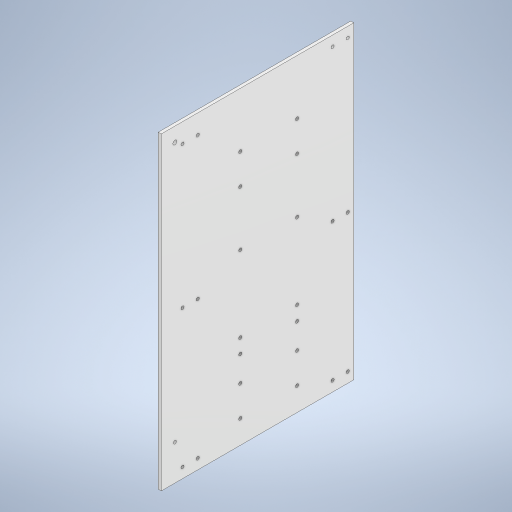
# Autodesk Inventor part: BP_Exterior-Right
Saved by Autodesk Inventor 2024.3 (Build 283343000, 343)
## iProperties
Created: 2025-04-22
Part Number: BP_Exterior-Right
Material: PBT プラスチック
Document SubType Name: Modeling
Designer: ngt-a
Density: 1.31 g/cm^3
Appearance: 滑らか - 白
Mass: 218.125 g
Surface Area: 1149.08 cm^2
Volume: 166.508 cm^3
Author: ngt-a
Autodesk Inventor part; units mm, degrees
ref_plane "YZ Plane" through (0, 0, 0) normal (1, 0, 0) x (0, 1, 0)
ref_plane "XZ Plane" through (0, 0, 0) normal (0, 1, 0) x (-1, 0, 0)
ref_plane "XY Plane" through (0, 0, 0) normal (0, 0, 1) x (1, 0, 0)
sketch "スケッチ1" plane through (0, 0, 0) normal (1, 0, 0) x (0, 1, 0)
  line L0 (75, 87.5) -> (-75, 87.5)
  line L1 (-75, 87.5) -> (-75, -87.5)
  line L2 (-75, -87.5) -> (75, -87.5)
  line L3 (75, -87.5) -> (75, 87.5)
  line L4 (75, 87.5) -> (-75, -87.5) construction
  line L5 (-75, 87.5) -> (75, -87.5) construction
  point P0 (0, 0)
  dimension "d0" = 150
  dimension "d1" = 175
  constraints: 12 end point, 2 midpoint, 2 parallel, 1 horizontal, 1 perpendicular
  measures "d0" distance of L1.end L2.end
  measures "d1" distance of L2.end L0.start
extrude "押し出し1" add sketch "スケッチ1" along normal blind 3
sketch "スケッチ2" plane through (3, 0, 0) normal (1, 0, 0) x (0, 0, -1)
  circle A0 centre (81.5, 66) radius 1.5
  circle A1 centre (66.5, 66) radius 1.5
  line L0 (87.5, -75) -> (87.5, 75) projected
  line L1 (87.5, 75) -> (-87.5, 75) projected
  line L2 (-87.5, 75) -> (-87.5, -75) projected
  line L3 (-87.5, 0) -> (87.5, 0)
  circle A2 centre (66.5, -70) radius 1.5
  circle A3 centre (81.5, -70) radius 1.5
  line L4 (-87.5, -75) -> (87.5, -75) projected
  point P0 (0, 0)
  dimension "d4" = 3
  dimension "d5" = 6
  dimension "d7" = 15
  dimension "d9" = 3
  dimension "d20" = 3
  dimension "d21" = 3
  dimension "d22" = 6
  dimension "d23" = 15
  dimension "d24" = 5
  dimension "d25" = 5
  dimension "d66" = 141
  dimension "d67" = 141
  constraints: 4 centre point, 2 end point, 2 midpoint
  measures "d4" diameter of A0
  measures "d5" distance from line of L0 A0.centre
  measures "d7" distance of A0.centre A1.centre
  measures "d9" diameter of A1
  measures "d20" diameter of A2
  measures "d21" diameter of A3
  measures "d22" distance from line of L0 A3.centre
  measures "d23" distance of A3.centre A2.centre
  measures "d24" distance from line of L4 A3.centre
  measures "d25" distance from line of A2.centre L4
  measures "d66" distance from line of L4 A0.centre
  measures "d67" distance from line of L4 A1.centre
extrude "押し出し2" cut sketch "スケッチ2" against normal through all contours A0 | A1 | A2 | A3
sketch "スケッチ3" plane through (0, 0, 0) normal (-1, 0, 0) x (0, 0, 1)
  circle A0 centre (81.5, 66) radius 1.5
  circle A1 centre (66.5, 66) radius 1.5
  line L0 (87.5, 75) -> (87.5, -75) projected
  line L1 (-87.5, 75) -> (87.5, 75) projected
  line L2 (-87.5, -75) -> (-87.5, 75) projected
  line L3 (-87.5, 0) -> (87.5, 0)
  circle A2 centre (81.5, -70) radius 1.5
  circle A3 centre (66.5, -70) radius 1.5
  line L4 (87.5, -75) -> (-87.5, -75) projected
  point P0 (0, 0)
  dimension "d12" = 6
  dimension "d13" = 3
  dimension "d14" = 15
  dimension "d15" = 3
  dimension "d26" = 3
  dimension "d27" = 3
  dimension "d28" = 15
  dimension "d29" = 6
  dimension "d30" = 5
  dimension "d31" = 5
  dimension "d64" = 141
  dimension "d65" = 141
  constraints: 4 centre point, 2 end point, 2 midpoint
  measures "d12" distance from line of L0 A0.centre
  measures "d13" diameter of A1
  measures "d14" distance of A0.centre A1.centre
  measures "d15" diameter of A0
  measures "d26" diameter of A3
  measures "d27" diameter of A2
  measures "d28" distance of A2.centre A3.centre
  measures "d29" distance from line of L0 A2.centre
  measures "d30" distance from line of L4 A2.centre
  measures "d31" distance from line of L4 A3.centre
  measures "d64" distance from line of L4 A1.centre
  measures "d65" distance from line of L4 A0.centre
sketch "スケッチ6" plane through (3, 0, 0) normal (1, 0, 0) x (0, 0, -1)
  circle A0 centre (-24.5, -57) radius 1.5
  circle A1 centre (31.5, -57) radius 1.5
  circle A2 centre (-24.5, -27) radius 1.5
  circle A3 centre (31.5, -27) radius 1.5
  line L0 (-87.5, -75) -> (87.5, -75) projected
  line L1 (-87.5, 75) -> (-87.5, -75) projected
  line L2 (87.5, -75) -> (87.5, 75) projected
  point P0 (0, 0)
  dimension "d32" = 3
  dimension "d33" = 3
  dimension "d34" = 3
  dimension "d35" = 18
  dimension "d36" = 18
  dimension "d38" = 30
  dimension "d43" = 3
  dimension "d46" = 56
  dimension "d47" = 56
  dimension "d50" = 56
  dimension "d51" = 56
  constraints: 4 centre point
  measures "d32" diameter of A2
  measures "d33" diameter of A0
  measures "d34" diameter of A1
  measures "d35" distance from line of L0 A0.centre
  measures "d36" distance from line of L0 A1.centre
  measures "d38" distance of A1.centre A3.centre
  measures "d43" diameter of A3
  measures "d46" distance of A3.centre A2.centre
  measures "d47" distance of A1.centre A0.centre
  measures "d50" distance from line of L2 A3.centre
  measures "d51" distance from line of L2 A1.centre
extrude "押し出し4" cut sketch "スケッチ6" against normal through all
sketch "スケッチ7" plane through (0, -75, 87.5) normal (0, 0, 1) x (1, 0, 0)
  line L0 (0, 150) -> (3, 150) projected
  line L1 (0, 0) -> (3, 0) projected
  line L2 (0, 150) -> (3, 150)
  line L3 (3, 150) -> (3, 0)
  line L4 (3, 0) -> (0, 0)
  line L5 (0, 0) -> (0, 150)
  point P0 (0, 75)
  constraints: 8 end point, 2 parallel, 1 horizontal, 1 perpendicular
extrude "押し出し5" add sketch "スケッチ7" along normal blind 10
sketch "スケッチ9" plane through (0, -75, -87.5) normal (0, -1, 0) x (1, 0, 0)
  line L0 (3, 0) -> (3, 185) projected
  line L1 (0, 185) -> (0, 0) projected
  line L2 (3, 18) -> (0, 18)
  line L3 (0, 18) -> (0, 43)
  line L4 (0, 43) -> (3, 43)
  line L5 (3, 43) -> (3, 18)
  line L6 (0, 142) -> (3, 142)
  line L7 (3, 142) -> (3, 167)
  line L8 (3, 167) -> (0, 167)
  line L9 (0, 167) -> (0, 142)
  line L10 (0, 0) -> (3, 0) projected
  line L11 (0, 185) -> (3, 185) projected
  point P0 (0, 87.5)
  point P1 (1.5, 185)
  point P2 (0, 167)
  point P3 (3, 142)
  point P4 (3, 43)
  point P5 (0, 18)
  dimension "d58" = 18
  dimension "d59" = 25
  dimension "d60" = 18
  dimension "d61" = 25
  constraints: 16 end point, 4 parallel, 4 point on line, 2 horizontal, 2 perpendicular, 1 midpoint
  measures "d58" distance between parallel lines of L2 L10
  measures "d59" distance between parallel lines of L2 L4
  measures "d60" distance from line of point (1.5, 185) L8
  measures "d61" distance between parallel lines of L8 L6
extrude "押し出し7" add sketch "スケッチ9" along normal blind 5
sketch "スケッチ10" plane through (0, 75, -87.5) normal (0, 1, 0) x (1, 0, 0)
  line L0 (0, 0) -> (0, -185) projected
  line L1 (3, 0) -> (3, -185) projected
  line L2 (0, 0) -> (3, 0)
  line L3 (3, 0) -> (3, -185)
  line L4 (3, -185) -> (0, -185)
  line L5 (0, -185) -> (0, 0)
  point P0 (0, -87.5)
  point P1 (3, 0)
  point P2 (0, -185)
  constraints: 8 end point, 2 parallel, 1 horizontal, 1 perpendicular
extrude "押し出し8" add sketch "スケッチ10" along normal blind 150
sketch "スケッチ11" plane through (3, 0, 0) normal (1, 0, 0) x (0, 0, -1)
  line L0 (44.5, -75) -> (-54.5, -75) projected
  line L1 (-54.5, -75) -> (44.5, -75)
  line L2 (44.5, -75) -> (44.5, -6)
  line L3 (44.5, -6) -> (-54.5, -6)
  line L4 (-54.5, -6) -> (-54.5, -75)
  line L5 (-54.5, -6) -> (44.5, -6)
  line L6 (44.5, -6) -> (44.5, 123)
  line L7 (44.5, 123) -> (-54.5, 123)
  line L8 (-54.5, 123) -> (-54.5, -6)
  circle A0 centre (-24.5, 87) radius 1.5
  circle A1 centre (31.5, 87) radius 1.5
  circle A2 centre (31.5, 12) radius 1.5
  circle A3 centre (-24.5, 12) radius 1.5
  line L9 (-54.5, 123) -> (44.5, 123)
  line L10 (44.5, 123) -> (44.5, 192)
  line L11 (44.5, 192) -> (-54.5, 192)
  line L12 (-54.5, 192) -> (-54.5, 123)
  circle A4 centre (31.5, 141) radius 1.5
  circle A5 centre (-24.5, 141) radius 1.5
  circle A6 centre (-24.5, 171) radius 1.5
  circle A7 centre (31.5, 171) radius 1.5
  point P0 (0, 0)
  point P1 (-5, -75)
  dimension "d70" = 69
  dimension "d71" = 129
  dimension "d72" = 3
  dimension "d73" = 3
  dimension "d74" = 30
  dimension "d75" = 13
  dimension "d89" = 3
  dimension "d90" = 3
  dimension "d136" = 69
  dimension "d137" = 18
  dimension "d138" = 18
  dimension "d139" = 75
  dimension "d140" = 75
  dimension "d141" = 18
  dimension "d142" = 18
  dimension "d143" = 3
  dimension "d144" = 3
  dimension "d145" = 30
  dimension "d146" = 30
  dimension "d147" = 3
  dimension "d148" = 3
  constraints: 24 end point, 8 centre point, 6 parallel, 3 horizontal, 3 perpendicular, 1 midpoint
  measures "d70" distance of L1.end L2.end
  measures "d71" distance of L5.end L6.end
  measures "d72" diameter of A0
  measures "d73" diameter of A1
  measures "d74" distance from line of A0.centre L8
  measures "d75" distance from line of L6 A1.centre
  measures "d89" diameter of A3
  measures "d90" diameter of A2
  measures "d136" distance of L9.end L10.end
  measures "d137" distance from line of L3 A3.centre
  measures "d138" distance from line of L3 A2.centre
  measures "d139" distance of A3.centre A0.centre
  measures "d140" distance of A2.centre A1.centre
  measures "d141" distance from line of L7 A4.centre
  measures "d142" distance from line of L7 A5.centre
  measures "d143" diameter of A5
  measures "d144" diameter of A4
  measures "d145" distance of A4.centre A7.centre
  measures "d146" distance of A5.centre A6.centre
  measures "d147" diameter of A6
  measures "d148" diameter of A7
extrude "押し出し9" cut sketch "スケッチ11" against normal blind 10 contours A0 | A1 | A2 | A3 | A4 | A5 | A6 | A7
extrude "押し出し10" cut sketch "スケッチ3" against normal blind 10 contours A0 | A1 | A2 | A3
sketch "スケッチ12" plane through (3, 0, 0) normal (1, 0, 0) x (0, 0, -1)
  circle A0 centre (-24.5, -2) radius 1.5
  line L0 (44.5, -75) -> (-54.5, -75) projected
  line L1 (-54.5, -75) -> (44.5, -75)
  line L2 (44.5, -75) -> (44.5, 118.2997)
  line L3 (44.5, 118.2997) -> (-54.5, 118.2997)
  line L4 (-54.5, 118.2997) -> (-54.5, -75)
  circle A1 centre (31.5, -2) radius 1.5
  circle A2 centre (-24.5, -57) radius 1.5 projected
  circle A3 centre (31.5, -57) radius 1.5 projected
  point P0 (0, 0)
  dimension "d93" = 30
  dimension "d94" = 3
  dimension "d95" = 13
  dimension "d96" = 3
  dimension "d97" = 55
  dimension "d98" = 55
  constraints: 8 end point, 2 centre point, 2 parallel, 1 horizontal, 1 perpendicular
  measures "d93" distance from line of A0.centre L4
  measures "d94" diameter of A0
  measures "d95" distance from line of L2 A1.centre
  measures "d96" diameter of A1
  measures "d97" distance of A2.centre A0.centre
  measures "d98" distance of A3.centre A1.centre
extrude "押し出し11" cut sketch "スケッチ12" against normal blind 10 contours A0 | A1
sketch "スケッチ13" plane through (0, 0, 0) normal (-1, 0, 0) x (0, 0, 1)
  circle A0 centre (-81.5, 66) radius 1.5 projected
  circle A1 centre (-81.5, 66) radius 3
  circle A2 centre (-66.5, 66) radius 1.5 projected
  circle A3 centre (-66.5, 66) radius 3
  circle A4 centre (66.5, 66) radius 1.5 projected
  circle A5 centre (66.5, 66) radius 3
  circle A6 centre (81.5, 66) radius 1.5 projected
  circle A7 centre (81.5, 66) radius 3
  circle A8 centre (-81.5, -70) radius 1.5 projected
  circle A9 centre (-81.5, -70) radius 3
  circle A10 centre (-66.5, -70) radius 1.5 projected
  circle A11 centre (-66.5, -70) radius 3
  circle A12 centre (66.5, -70) radius 1.5 projected
  circle A13 centre (66.5, -70) radius 3
  circle A14 centre (81.5, -70) radius 1.5 projected
  circle A15 centre (81.5, -70) radius 3
  point P0 (0, 0)
  dimension "d101" = 6
  dimension "d102" = 6
  dimension "d103" = 6
  dimension "d104" = 6
  dimension "d105" = 6
  dimension "d106" = 6
  dimension "d107" = 6
  dimension "d108" = 6
  constraints: 8 centre point, 8 coincident
  measures "d101" diameter of A9
  measures "d102" diameter of A11
  measures "d103" diameter of A15
  measures "d104" diameter of A13
  measures "d105" diameter of A1
  measures "d106" diameter of A3
  measures "d107" diameter of A5
  measures "d108" diameter of A7
extrude "押し出し12" cut sketch "スケッチ13" against normal blind 1
sketch "スケッチ14" plane through (0, 0, 0) normal (-1, 0, 0) x (0, 0, 1)
  circle A0 centre (66.5, 206) radius 1.5
  circle A1 centre (81.5, 206) radius 1.5
  line L0 (97.5, -80) -> (97.5, 225) projected
  line L1 (-87.5, 225) -> (97.5, 225) projected
  point P0 (0, 0)
  point P1 (97.5, -75)
  dimension "d111" = 16
  dimension "d112" = 15
  dimension "d113" = 19
  dimension "d114" = 19
  dimension "d115" = 3
  dimension "d116" = 3
  constraints: 2 centre point
  measures "d111" distance from line of L0 A1.centre
  measures "d112" distance of A1.centre A0.centre
  measures "d113" distance from line of A1.centre L1
  measures "d114" distance from line of A0.centre L1
  measures "d115" diameter of A1
  measures "d116" diameter of A0
extrude "押し出し13" cut sketch "スケッチ14" against normal blind 10
sketch "スケッチ15" plane through (0, 0, 0) normal (-1, 0, 0) x (0, 0, 1)
  circle A0 centre (66.5, 206) radius 1.5 projected
  circle A1 centre (66.5, 206) radius 3
  circle A2 centre (81.5, 206) radius 1.5 projected
  circle A3 centre (81.5, 206) radius 3
  point P0 (0, 0)
  dimension "d119" = 6
  dimension "d120" = 6
  constraints: 2 centre point, 2 coincident
  measures "d119" diameter of A1
  measures "d120" diameter of A3
extrude "押し出し14" cut sketch "スケッチ15" against normal blind 1
sketch "スケッチ16" plane through (0, 0, 0) normal (-1, 0, 0) x (0, 0, 1)
  circle A0 centre (-81.5, 215) radius 1.5
  circle A1 centre (-66.5, 215) radius 1.5
  line L0 (-87.5, -75) -> (-87.5, 225) projected
  line L1 (-87.5, 225) -> (97.5, 225) projected
  point P0 (0, 0)
  dimension "d123" = 6
  dimension "d124" = 10
  dimension "d126" = 10
  dimension "d127" = 3
  dimension "d128" = 3
  dimension "d131" = 15
  constraints: 2 centre point
  measures "d123" distance from line of A0.centre L0
  measures "d124" distance from line of A0.centre L1
  measures "d126" distance from line of L1 A1.centre
  measures "d127" diameter of A0
  measures "d128" diameter of A1
  measures "d131" distance of A1.centre A0.centre
extrude "押し出し15" cut sketch "スケッチ16" against normal through all
sketch "スケッチ17" plane through (0, 0, 0) normal (-1, 0, 0) x (0, 0, 1)
  circle A0 centre (-81.5, 215) radius 1.5 projected
  circle A1 centre (-81.5, 215) radius 3
  circle A2 centre (-66.5, 215) radius 1.5 projected
  circle A3 centre (-66.5, 215) radius 3
  point P0 (0, 0)
  dimension "d132" = 6
  dimension "d133" = 6
  constraints: 2 centre point, 2 coincident
  measures "d132" diameter of A1
  measures "d133" diameter of A3
extrude "押し出し16" cut sketch "スケッチ17" against normal blind 1
sketch "スケッチ19" plane through (0, -75, 97.5) normal (0, 0, 1) x (1, 0, 0)
  line L0 (3, 0) -> (3, 300) projected
  line L1 (0, 0) -> (3, 0) projected
  line L2 (3, 300) -> (0, 300)
  line L3 (0, 300) -> (0, 0)
  line L4 (0, 0) -> (3, 0)
  line L5 (3, 0) -> (3, 300)
  point P0 (0, 75)
  constraints: 8 end point, 2 parallel, 1 horizontal, 1 perpendicular
extrude "押し出し17" add sketch "スケッチ19" along normal blind 5
sketch "スケッチ18" plane through (0, 0, 0) normal (-1, 0, 0) x (0, 0, 1)
  line L0 (77.5, 225) -> (100.5, 225)
  line L1 (100.5, 225) -> (100.5, -75)
  line L2 (100.5, -75) -> (77.5, -75)
  line L3 (77.5, -75) -> (77.5, 225)
  line L4 (102.5, 225) -> (102.5, -75) projected
  circle A0 centre (89, -45) radius 1.5
  circle A1 centre (89, 211) radius 2
  line L5 (102.5, -75) -> (79.5, -75) projected
  point P0 (0, 0)
  point P1 (91, -75)
  dimension "d149" = 23
  dimension "d153" = 2
  dimension "d154" = 14
  dimension "d155" = 3
  dimension "d156" = 30
  dimension "d157" = 4
  dimension "d160" = 11.5
  dimension "d161" = 11.5
  constraints: 8 end point, 2 centre point, 2 parallel, 1 horizontal, 1 midpoint, 1 perpendicular
  measures "d149" distance between parallel lines of L1 L3
  measures "d153" distance between parallel lines of L4 L1
  measures "d154" distance from line of A1.centre L0
  measures "d155" diameter of A0
  measures "d156" vertical distance of point (91, -75) A0.centre
  measures "d157" diameter of A1
  measures "d160" distance from line of L1 A1.centre
  measures "d161" distance from line of L1 A0.centre
extrude "押し出し18" cut sketch "スケッチ18" against normal blind 5 contours A0 | A1
sketch "スケッチ20" plane through (0, -75, 97.5) normal (0, -1, 0) x (1, 0, 0)
  line L0 (3, 0) -> (0, 0) projected
  line L1 (3, 0) -> (3, 5) projected
  line L2 (0, 5) -> (3, 5) projected
  line L3 (0, 0) -> (0, 5) projected
  point P0 (0, -97.5)
extrude "押し出し19" add sketch "スケッチ20" along normal blind 5
